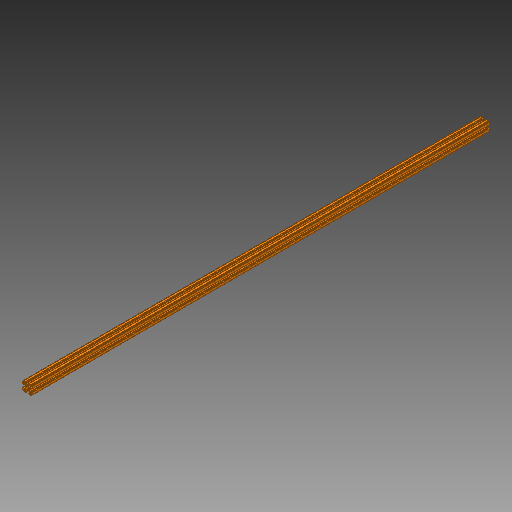
# Autodesk Inventor part: Rail
Saved by Autodesk Inventor 2017 SP1 (Build 210196100, 196)
## iProperties
Created: 2018-01-18
Part Number: Rail
Material: Aluminum 6061
Document SubType Name: Modeling
Designer: Ben
Density: 2.7 g/cm^3
Appearance: Orange
Mass: 865.797 g
Surface Area: 3011.97 cm^2
Volume: 320.666 cm^3
Author: Ben
Autodesk Inventor part; units mm, degrees
ref_plane "YZ Plane" through (0, 0, 0) normal (1, 0, 0) x (0, 1, 0)
ref_plane "XZ Plane" through (0, 0, 0) normal (0, 1, 0) x (-1, 0, 0)
ref_plane "XY Plane" through (0, 0, 0) normal (0, 0, 1) x (1, 0, 0)
sketch "Sketch1" plane through (0, 0, 0) normal (0, 0, 1) x (1, 0, 0)
  arc A0 (0, 2.032) -> (-2.032, 0) centre (0, 0) ccw
  line L0 (-4.24, 12.6256) -> (-2.9954, 11.381)
  line L1 (-3.175, 10.9474) -> (-4.7625, 10.9474)
  line L2 (-4.7625, 10.9474) -> (-4.7625, 7.2898)
  line L3 (-4.4196, 12.7) -> (-10.1166, 12.7)
  arc A1 (-8.0882, 8.0882) -> (-7.6411, 8.7636) centre (-9.525, 9.525) ccw construction
  arc A2 (-10.1166, 12.7) -> (-9.9809, 11.5052) centre (-10.1166, 12.0949) ccw
  line L4 (-10.5445, 11.667) -> (-11.1057, 11.1057) construction
  arc A3 (-4.7625, 7.2898) -> (-2.5781, 5.1054) centre (-2.5781, 7.2898) ccw
  arc A4 (-2.5781, 5.1054) -> (-1.0541, 3.5814) centre (-1.0541, 5.1054) ccw
  line L5 (-1.0541, 3.5814) -> (0, 3.5814)
  line L6 (-2.5781, 5.1054) -> (0, 5.1054) construction
  line L7 (0, 0) -> (-11.1057, 11.1057) construction
  line L8 (-12.6256, 4.24) -> (-11.381, 2.9954)
  line L9 (-10.9474, 3.175) -> (-10.9474, 4.7625)
  line L10 (-10.9474, 4.7625) -> (-7.2898, 4.7625)
  line L11 (-12.7, 4.4196) -> (-12.7, 10.1166)
  arc A5 (-11.5052, 9.9809) -> (-8.7636, 7.6411) centre (-9.525, 9.525) ccw
  arc A6 (-11.5052, 9.9809) -> (-12.7, 10.1166) centre (-12.0949, 10.1166) ccw
  arc A7 (-5.1054, 2.5781) -> (-7.2898, 4.7625) centre (-7.2898, 2.5781) ccw
  arc A8 (-3.5814, 1.0541) -> (-5.1054, 2.5781) centre (-5.1054, 1.0541) ccw
  line L12 (-3.5814, 1.0541) -> (-3.5814, 0)
  line L13 (0, 3.5814) -> (0, 2.032)
  line L14 (-3.5814, 0) -> (-2.032, 0)
  arc A9 (-3.175, 10.9474) -> (-2.9954, 11.381) centre (-3.175, 11.2014) ccw
  arc A10 (-11.381, 2.9954) -> (-10.9474, 3.175) centre (-11.2014, 3.175) ccw
  arc A11 (-12.7, 4.4196) -> (-12.6256, 4.24) centre (-12.446, 4.4196) ccw
  arc A12 (-4.24, 12.6256) -> (-4.4196, 12.7) centre (-4.4196, 12.446) ccw
  line L15 (-2.921, 11.2014) -> (0, 11.2014) construction
  line L16 (-8.7636, 7.6411) -> (-7.6411, 6.5185)
  line L17 (-7.6411, 6.5185) -> (-6.5185, 7.6411)
  line L18 (-6.5185, 7.6411) -> (-7.6411, 8.7636)
  arc A13 (-8.7636, 7.6411) -> (-8.0882, 8.0882) centre (-9.525, 9.525) ccw construction
  arc A14 (-7.6411, 8.7636) -> (-9.9809, 11.5052) centre (-9.525, 9.525) ccw
  point P0 (-4.3144, 12.7)
  point P1 (-2.5618, 10.9474)
  point P2 (-12.7, 4.3144)
  point P3 (-10.9474, 2.5618)
  point P4 (-7.0798, 7.0798)
  dimension "d0" = 4.064
  dimension "d1" = 45
  dimension "d10" = 0.7937
  dimension "d13" = 2.5781
  dimension "d14" = 1.7526
  dimension "d21" = 1.5494
  dimension "d23" = 0.254
  dimension "d24" = 2.921
  dimension "d30" = 12.7
  dimension "d32" = 9.525
  dimension "d33" = 4.7625
  dimension "d34" = 1.524
  constraints: 39 end point, 32 point on circle, 17 point on line, 15 centre point, 13 tangent, 12 symmetric about line, 6 horizontal, 5 perpendicular, 4 equal radius, 2 parallel, 1 coincident, 1 midpoint, 1 vertical, 5 other
  measures "d0" diameter of A0
  measures "d1" angle of L1 L0
  measures "d10" distance of L4.end L4.start
  measures "d13" distance of L6.start L6.end
  measures "d14" distance between parallel lines of L3 L1
  measures "d21" distance of L5.end L13.end
  measures "d23" radius of A9
  measures "d24" distance of L15.start L15.end
  measures "d30" distance from line of point (0, 0) L11
  measures "d32" horizontal distance of point (0, 0) A1.centre
  measures "d33" distance between parallel lines of L13 L2
  measures "d34" distance between parallel lines of L6 L5
extrude "Extrusion1" add sketch "Sketch1" along normal mid plane 1219.2
pattern_circular "Circular Pattern1" count 4 over 360 about axis through (0, 0, -10) along (0, 0, 1) of "Extrusion1"
body "Solid1"
